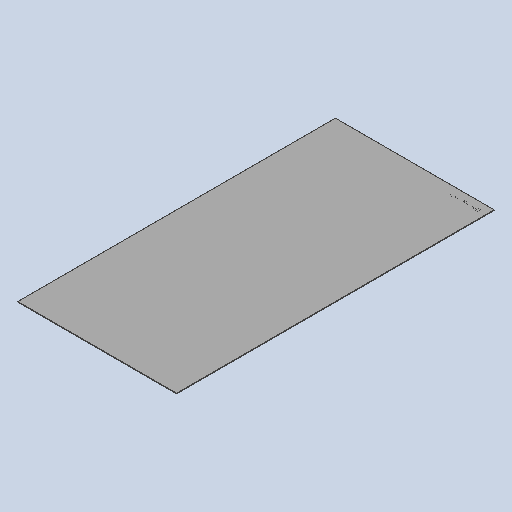
# Autodesk Inventor part: TRM 019 tray
Saved by Autodesk Inventor 2025 (Build 290162010, 162A)
## iProperties
Created: 2024-08-07
Part Number: TRM 019 tray
Material: AISI 304
Document SubType Name: Sheet Metal
Designer: pokla
Density: 8.02768 g/cm^3
Flat Pattern Width: 50 cm
Flat Pattern Length: 100 cm
Flat Pattern Area: 5000 cm^2
Sheet Metal Rule: AISI304 2mm Die16
Sheet Metal Width: 500,000 mm
Sheet Metal Length: 1000,000 mm
Sheet Metal Area: 500000,000 mm^2
Appearance: Default
Stock Number: ТРМ 019 лоток
Author: pokla
Autodesk Inventor part; units mm, degrees
ref_plane "YZ Plane" through (0, 0, 0) normal (1, 0, 0) x (0, 1, 0)
ref_plane "XZ Plane" through (0, 0, 0) normal (0, 1, 0) x (-1, 0, 0)
ref_plane "XY Plane" through (0, 0, 0) normal (0, 0, 1) x (1, 0, 0)
sketch "Sketch1" plane through (0, 0, 0) normal (0, 0, 1) x (1, 0, 0)
  line L0 (-250, -500) -> (250, -500)
  line L1 (250, -500) -> (250, 500)
  line L2 (250, 500) -> (-250, 500)
  line L3 (-250, 500) -> (-250, -500)
  line L4 (-250, -500) -> (250, 500) construction
  line L5 (250, -500) -> (-250, 500) construction
  point P0 (0, 0)
  dimension "d0" = 500
  dimension "d1" = 1000
  measures "d0" distance of L2.end L1.end
  measures "d1" distance of L1.end L0.end
extrude "Plate1" add sketch "Sketch1" along normal blind 2
sketch "Sketch2" plane through (0, 0, 0) normal (0, 0, -1) x (-1, 0, 0)
  line L0 (-230, 480) -> (-30, 480) construction
  line L1 (-30, 480) -> (-30, 460) construction
  line L2 (-30, 460) -> (-230, 460) construction
  line L3 (-230, 460) -> (-230, 480) construction
  line L4 (-250, 500) -> (250, 500) projected
  line L5 (-250, -500) -> (-250, 500) projected
  point P0 (0, 0)
  point P1 (-48, 100)
  point P2 (250, 500)
  point P3 (-50, 98)
  dimension "d6" = 200
  dimension "d9" = 20
  dimension "d10" = 20
  dimension "d11" = 20
  constraints: 4 other
  measures "d6" distance of L0.start L0.end
  measures "d9" distance of L0.end L1.end
  measures "d11" length of L3
mark "Mark1"
equation "\"d2\" = Thickness"
equation "\"BendReliefWidth\" = Thickness"
equation "\"BendReliefDepth\" = 0.5 * Thickness"
equation "\"CornerReliefSize\" = 4 * Thickness"
equation "\"MinimumRemnant\" = 2 * Thickness"
equation "\"TransitionRadius\" = BendRadius"
equation "\"JacobiRadiusSize\" = BendRadius"
equation "\"GapSize\" = Thickness"
equation "\"Thickness\" = 2"
equation "\"BendRadius\" = 2.75"
body "Solid1"
